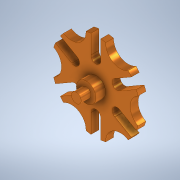
# Autodesk Inventor part: genevawheel
Saved by Autodesk Inventor 2022 (Build 260153000, 153)
## iProperties
Created: 2023-01-28
Part Number: genevawheel
Material: Gold
Document SubType Name: Modeling
Designer: karee
Density: 19.3 g/cm^3
Appearance: Metal 1600F Hot
Author: karee
Autodesk Inventor part; units mm, degrees
ref_plane "YZ Plane" through (0, 0, 0) normal (1, 0, 0) x (0, 1, 0)
ref_plane "XZ Plane" through (0, 0, 0) normal (0, 1, 0) x (-1, 0, 0)
ref_plane "XY Plane" through (0, 0, 0) normal (0, 0, 1) x (1, 0, 0)
sketch "Sketch1" plane through (0, 0, 0) normal (0, 0, 1) x (1, 0, 0)
  point P0 (0, 0)
sketch "Sketch2" plane through (0, 0, 0) normal (0, 0, 1) x (1, 0, 0)
  arc A0 (17.3205, 10) -> (24.5524, 8.4282) centre (21.6506, 12.5) ccw
  line L0 (24.5524, 8.4282) -> (41.2206, 18.0516)
  line L1 (0, 0) -> (17.3205, 10)
  arc A1 (43, 13.2665) -> (41.2206, 18.0516) centre (0, 0) ccw
  arc A2 (43, 13.2665) -> (35, 0) centre (50, 0) ccw
  line L2 (0, 0) -> (35, 0)
  dimension "d4" = 5
  dimension "d5" = 25
  dimension "d6" = 30
  dimension "d7" = 50
  dimension "d8" = 45
  dimension "d9" = 15
  constraints: 6 end point, 6 point on circle, 3 centre point, 1 coincident, 1 parallel
  measures "d4" radius of A0
  measures "d5" distance of A0.centre point (0, 0)
  measures "d6" angle of L1 L2
  measures "d7" distance of point (0, 0) A2.centre
  measures "d8" radius of A1
  measures "d9" radius of A2
extrude "Extrusion1" add sketch "Sketch2" along normal blind 8
mirror "Mirror1" about plane through (17.3205, 10, 0) normal (-0.5, 0.8660254, 0) of "Extrusion1"
pattern_circular "Circular Pattern1" count 6 over 360 about axis through (0, 0, 0) along (0, 0, 1) of "Extrusion1", "Mirror1"
sketch "Sketch3" plane through (0, 0, 8) normal (0, 0, 1) x (1, 0, 0)
  circle A0 centre (0, 0) radius 10
  dimension "d15" = 10
  constraints: 1 centre point, 1 coincident
  measures "d15" radius of A0
extrude "Extrusion2" add sketch "Sketch3" along normal blind 10
sketch "Sketch4" plane through (0, 0, 18) normal (0, 0, 1) x (1, 0, 0)
  circle A0 centre (0, 0) radius 5
  dimension "d18" = 5
  constraints: 1 centre point, 1 coincident
  measures "d18" radius of A0
extrude "Extrusion3" add sketch "Sketch4" along normal blind 10
body "Solid1"
